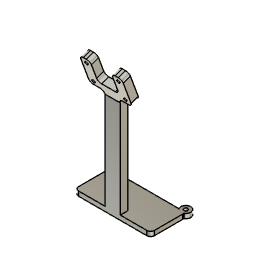
cam mount (Autodesk Fusion 360 design; units mm, degrees)
Autodesk Fusion 360 part; units mm, degrees
note: some values were not read from the file. Chosen so that the rebuilt part matches the saved one: which bodies a step acts on; which face or edge a step refers to. Set by a fixed rule: which sketch regions a step uses.
sketch "Sketch1" plane through (0, 0, 0) normal (0, 0, 1) x (1, 0, 0)
  line L0 (-25, 25) -> (25, 25)
  line L1 (25, 25) -> (25, 2)
  line L2 (25, 2) -> (-25, 2)
  line L3 (-25, 2) -> (-25, 25)
  line L4 (-25, 25) -> (-23.4, 25)
  line L5 (25, 25) -> (23.4, 25)
  line L6 (-21.7878, 23.1884) -> (-25.0122, 23.1884)
  line L7 (-25.0122, 23.1884) -> (-25.0122, 26.8116)
  line L8 (-21.7878, 26.8116) -> (-21.7878, 23.1884)
  line L9 (-21.7878, 23.1884) -> (-25.0122, 26.8116) construction
  line L10 (-25.0122, 23.1884) -> (-21.7878, 26.8116) construction
  circle A0 centre (-23.4, 26.8116) radius 1.25
  circle A1 centre (-23.4, 26.8116) radius 3.25
  line L11 (0, 25) -> (0, 2) construction
  circle A2 centre (23.4, 26.8116) radius 3.25
  circle A3 centre (23.4, 26.8116) radius 1.25
  line L12 (21.7878, 26.8116) -> (21.7878, 23.1884)
  line L13 (25.0122, 23.1884) -> (25.0122, 26.8116)
  line L14 (21.7878, 23.1884) -> (25.0122, 23.1884)
  point P0 (-23.4, 25)
  dimension "d1" = 50
  dimension "d2" = 23
  dimension "d3" = 1.6
  dimension "d4" = 1.6
  dimension "d5" = 2.5
  dimension "d6" = 2
  constraint horizontal L0
  constraint vertical L1
  constraint horizontal L2
  constraint vertical L3
  constraint perpendicular L3 L4
  constraint perpendicular L1 L5
  constraint horizontal L6
  constraint perpendicular L6 L7
  constraint parallel L7 L8
  constraint coincident L9 P0
  constraint coincident L10 P0
  constraint coincident P0 L4.end
  constraint midpoint L0 L11.start
  constraint midpoint L2 L11.end
  constraint symmetric L6.start L11 L12.end
  constraint symmetric L6.end L11 L13.start
  constraint symmetric L7.end L11 L13.end
  constraint symmetric L8.start L11 L12.start
  constraint symmetric A0 L11 A3
  constraint symmetric A1 L11 A2
  measures "d1" distance of L0.start L0.end
  measures "d2" distance of L0.start L2.end
  measures "d3" distance of L0.start P0
  measures "d4" distance of L0.end L5.end
  measures "d5" diameter of A0
extrude "Extrude1" add sketch "Sketch1" along normal blind 3 contours L0 L3 L4 A1 | L0 L3 L4 L8 A1 | L3 L6 L8 A1 | L3 L6 L7 A1 | L0 L8 A1 | L0 L1 L2 L3 L6 L8 A1 A2 L12 L14 | L0 L1 L5 A2 | L0 A2 L12 | L0 L1 L5 A2 L12 | L1 A2 L12 L14 | L1 A2 L13 L14 | A0 | A3 makes body 1
sketch "Sketch2" plane through (0, 0, 3) normal (0, 0, 1) x (-1, 0, 0)
  line L0 (-25, -23.1884) -> (-25.0122, -23.1884)
  line L1 (-25.0122, -23.1884) -> (-25.0122, -23.9897)
  arc A0 (-25.0122, -23.9897) -> (-20.7017, -25) centre (-23.4, -26.8116) ccw
  line L2 (-20.7017, -25) -> (20.7017, -25)
  arc A1 (20.7017, -25) -> (25.0122, -23.9897) centre (23.4, -26.8116) ccw
  line L3 (25.0122, -23.9897) -> (25.0122, -23.1884)
  line L4 (25.0122, -23.1884) -> (25, -23.1884)
  line L5 (25, -23.1884) -> (25, -2)
  line L6 (25, -2) -> (-25, -2)
  line L7 (-25, -2) -> (-25, -23.1884)
  line L8 (5, -2) -> (-5, -2)
  line L9 (-5, -2) -> (-5, -7)
  line L10 (-5, -7) -> (5, -7)
  line L11 (5, -7) -> (5, -2)
  dimension "d35" = 5
  constraint horizontal L8
  constraint vertical L9
  constraint horizontal L10
  constraint vertical L11
  constraint coincident L6 L8.start
  measures "d35" distance of L8.start L10.end
extrude "Extrude3" add sketch "Sketch2" along normal blind 70 contours L6 L8 L9 L10 L11 bodies 1
sketch "Sketch3" plane through (0, 0, 73) normal (0, 0, 1) x (-1, 0, 0)
  line L0 (5, -7) -> (5, -2)
  line L1 (5, -2) -> (-5, -2)
  line L2 (-5, -2) -> (-5, -7)
  line L3 (-5, -7) -> (5, -7)
sketch "Sketch4" plane through (0, 2, 0) normal (0, -1, 0) x (1, 0, 0)
  line L0 (-25, 0) -> (25, 0)
  line L1 (25, 0) -> (25, 3)
  line L2 (25, 3) -> (5, 3)
  line L3 (5, 3) -> (5, 73)
  line L4 (5, 73) -> (-5, 73)
  line L5 (-5, 73) -> (-5, 3)
  line L6 (-5, 3) -> (-25, 3)
  line L7 (-25, 3) -> (-25, 0)
  line L8 (-14, 70) -> (14, 70)
  line L9 (14, 70) -> (14, 90)
  line L10 (14, 90) -> (-14, 90)
  line L11 (-14, 90) -> (-14, 70)
  circle A0 centre (-10.6096, 86.4224) radius 1.1
  circle A1 centre (10.3904, 86.4224) radius 1.1
  circle A2 centre (-10.6096, 72.9224) radius 1.1
  circle A3 centre (10.3904, 72.9224) radius 1.1
  dimension "d13" = 28
  dimension "d14" = 20
  dimension "d15" = 21
  dimension "d16" = 13.5
  dimension "d17" = 2.2
  dimension "d18" = 2.2
  dimension "d19" = 2.2
  dimension "d20" = 2.2
  constraint horizontal L8
  constraint vertical L9
  constraint horizontal L10
  constraint vertical L11
  measures "d13" distance of L8.start L8.end
  measures "d14" distance of L8.start L10.end
  measures "d15" distance of A2.centre A3.centre
  measures "d16" distance of A0.centre A2.centre
  measures "d17" diameter of A0
  measures "d18" diameter of A1
  measures "d19" diameter of A2
  measures "d20" diameter of A3
extrude "Extrude4" add sketch "Sketch4" against normal blind 5 contours L3 L4 L5 L8 L9 L10 L11 | L3 L4 L5 L8 bodies 1
sketch "Sketch5" plane through (0, 2, 0) normal (0, -1, 0) x (1, 0, 0)
  circle A0 centre (-10.6096, 86.4224) radius 1.1
  circle A1 centre (-10.6096, 72.9224) radius 1.1
  circle A2 centre (10.3904, 72.9224) radius 1.1
  circle A3 centre (10.3904, 86.4224) radius 1.1
  line L0 (5, 70) -> (14, 70)
  line L1 (14, 70) -> (14, 90)
  line L2 (14, 90) -> (-14, 90)
  line L3 (-14, 90) -> (-14, 70)
  line L4 (-14, 70) -> (-5, 70)
  line L5 (-5, 70) -> (-5, 3)
  line L6 (-5, 3) -> (-25, 3)
  line L7 (-25, 3) -> (-25, 0)
  line L8 (-25, 0) -> (25, 0)
  line L9 (25, 0) -> (25, 3)
  line L10 (25, 3) -> (5, 3)
  line L11 (5, 3) -> (5, 70)
  line L12 (-7, 90) -> (7, 90)
  line L13 (7, 90) -> (7, 75)
  line L14 (7, 75) -> (-7, 75)
  line L15 (-7, 75) -> (-7, 90)
  constraint horizontal L12
  constraint vertical L13
  constraint horizontal L14
  constraint vertical L15
  constraint coincident L2 L12.start
extrude "Extrude5" cut sketch "Sketch5" against normal blind 11 contours L2 L12 L13 L14 L15 bodies 1
fillet "Fillet1" radius 2.5 4 edges at (-14, 4.5, 90) (-14, 4.5, 70) (14, 4.5, 90) (14, 4.5, 70) on bodies 1
fillet "Fillet2" radius 2.5 2 edges at (7, 4.5, 90) (-7, 4.5, 90) on bodies 1
fillet "Fillet3" radius 2.5 2 edges at (7, 4.5, 75) (-7, 4.5, 75) on bodies 1
fillet "Fillet4" radius 2.5 2 edges at (-5, 4.5, 70) (5, 4.5, 70) on bodies 1
fillet "Fillet5" radius 2.5 2 edges at (-25, 2, 1.5) (25, 2, 1.5) on bodies 1
copy_body "Body->Comp1" bodies 1 removing the originals makes body 2 in component "Component"
sketch "Sketch6" plane through (0, 2, 0) normal (0, -1, 0) x (1, 0, 0)
  line L0 (22.5, 0) -> (22.5, 3)
  line L1 (22.5, 3) -> (5, 3)
  line L2 (5, 3) -> (5, 67.5)
  arc A0 (7.5, 70) -> (5, 67.5) centre (7.5, 67.5) ccw
  line L3 (7.5, 70) -> (11.5, 70)
  arc A1 (11.5, 70) -> (14, 72.5) centre (11.5, 72.5) ccw
  line L4 (14, 72.5) -> (14, 87.5)
  arc A2 (14, 87.5) -> (11.5, 90) centre (11.5, 87.5) ccw
  line L5 (11.5, 90) -> (9.5, 90)
  arc A3 (9.5, 90) -> (7, 87.5) centre (9.5, 87.5) ccw
  line L6 (7, 87.5) -> (7, 77.5)
  arc A4 (4.5, 75) -> (7, 77.5) centre (4.5, 77.5) ccw
  line L7 (4.5, 75) -> (-4.5, 75)
  arc A5 (-7, 77.5) -> (-4.5, 75) centre (-4.5, 77.5) ccw
  line L8 (-7, 77.5) -> (-7, 87.5)
  arc A6 (-7, 87.5) -> (-9.5, 90) centre (-9.5, 87.5) ccw
  line L9 (-9.5, 90) -> (-11.5, 90)
  arc A7 (-11.5, 90) -> (-14, 87.5) centre (-11.5, 87.5) ccw
  line L10 (-14, 87.5) -> (-14, 72.5)
  arc A8 (-14, 72.5) -> (-11.5, 70) centre (-11.5, 72.5) ccw
  line L11 (-11.5, 70) -> (-7.5, 70)
  arc A9 (-5, 67.5) -> (-7.5, 70) centre (-7.5, 67.5) ccw
  line L12 (-5, 67.5) -> (-5, 3)
  line L13 (-5, 3) -> (-22.5, 3)
  line L14 (-22.5, 3) -> (-22.5, 0)
  line L15 (-22.5, 0) -> (22.5, 0)
  circle A10 centre (10.3904, 72.9224) radius 1.1
  circle A11 centre (-10.6096, 72.9224) radius 1.1
  circle A12 centre (10.3904, 86.4224) radius 1.1
  circle A13 centre (-10.6096, 86.4224) radius 1.1
  line L16 (-5, 67) -> (5, 67)
  constraint coincident L12 L16.start
  constraint coincident L2 L16.end
  constraint perpendicular L2 L16
split "Split1" by curves path "Sketch6" along L16 bodies 2 makes body 3 at (-6.9006, 9.6667, 0) in component "Component"
sketch "Sketch7" plane through (-5, 0, 0) normal (-1, 0, 0) x (0, -1, 0)
  line L0 (-2, 67) -> (-7, 67)
  line L1 (-7, 67) -> (-7, 3)
  line L2 (-7, 3) -> (-2, 3)
  line L3 (-2, 3) -> (-2, 67)
sketch "Sketch8" plane through (-5, 0, 0) normal (-1, 0, 0) x (0, -1, 0)
move_body "Move1" bodies 2 to x (1, 0, 0) y (0, 0.939693, 0.34202) z (0, -0.34202, 0.939693) at (0, 23.036, 3.3566) in component "Component"
extrude "Extrude1'" add 1 faces at (-1.6667, 5.3333, 67) along direction (0, 0, 1) blind 2 on bodies 3 bodies 2 3 in component "Component"
sketch "Sketch13" plane through (-5, 0, 0) normal (-1, 0, 0) x (0, -1, 0)
  line L0 (-7, 69) -> (-7, 3)
  line L1 (-7, 3) -> (-2, 3)
  line L2 (-2, 3) -> (-2, 67)
  line L3 (-2, 67) -> (-1.829, 67.4698)
  line L4 (-1.829, 67.4698) -> (-6.5275, 69.1799)
  line L5 (-6.5275, 69.1799) -> (-6.5929, 69)
  line L6 (-6.5929, 69) -> (-7, 69)
  line L7 (-6.5929, 69) -> (-7, 68.4)
  constraint coincident L5.end L6.start
  constraint coincident L0 L7.end
extrude "Extrude2" cut sketch "Sketch13" against normal blind 14 contours L0 L6 L7 bodies 2 in component "Component"
extrude "Extrude3'" cut sketch "Sketch1" along normal blind 3 contours A3 bodies 2 in component "Component"
extrude "Extrude4'" cut sketch "Sketch1" along normal blind 3 contours A0 bodies 2 in component "Component"
component "Component" placed x (1, 0, 0) y (0, 1, 0) z (0, 0, 1) at (0, 0, 0)
